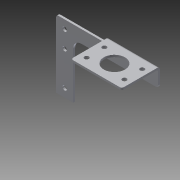
# Autodesk Inventor part: Circuit Breaker Mount
Saved by Autodesk Inventor 2013 (Build 170138000, 138)
## iProperties
Created: 2013-02-10
Part Number: Circuit Breaker Mount
Material: Aluminum 6061
Document SubType Name: Sheet Metal
Designer: Moses
Mass: 60.4905 g
Surface Area: 168.953 cm^2
Volume: 22.3212 cm^3
Density: 2.71 g/cm^3
Sheet Metal Rule: Default
Author: Moses
Autodesk Inventor part; units mm, degrees
ref_plane "YZ Plane" through (0, 0, 0) normal (1, 0, 0) x (0, 1, 0)
ref_plane "XZ Plane" through (0, 0, 0) normal (0, 1, 0) x (-1, 0, 0)
ref_plane "XY Plane" through (0, 0, 0) normal (0, 0, 1) x (1, 0, 0)
sketch "Sketch1" plane through (0, 0, 0) normal (0, 0, 1) x (1, 0, 0)
  line L0 (0, 0) -> (25.4, 0)
  line L1 (25.4, 0) -> (25.4, 50.8)
  line L2 (25.4, 50.8) -> (0, 50.8)
  line L3 (0, 50.8) -> (0, 0)
  line L4 (0, 25.4) -> (25.4, 25.4) construction
  line L5 (12.7, 38.1) -> (12.7, 12.7) construction
  circle A0 centre (12.7, 38.1) radius 3.302
  circle A1 centre (12.7, 12.7) radius 3.302
  line L6 (152.4, 50.8) -> (25.4, 50.8)
  line L7 (25.4, 31.75) -> (152.4, 31.75)
  line L8 (152.4, 31.75) -> (152.4, 50.8)
  line L9 (76.2, 50.8) -> (76.2, 53.975)
  line L10 (76.2, 53.975) -> (152.4, 53.975)
  line L11 (152.4, 53.975) -> (152.4, 50.8)
  line L12 (0, 0) -> (0, -50.8)
  line L13 (0, -50.8) -> (25.4, -50.8)
  line L14 (25.4, -50.8) -> (25.4, 0)
  line L15 (12.7, 12.7) -> (12.7, -38.1) construction
  circle A2 centre (12.7, -38.1) radius 3.302
  point P0 (12.7, 25.4)
  dimension "d0" = 25.4
  dimension "d2" = 6.604
  dimension "d3" = 6.604
  dimension "d4" = 50.8
  dimension "d5" = 25.4
  dimension "d6" = 127
  dimension "d7" = 19.05
  dimension "d8" = 76.2
  dimension "d9" = 3.175
  dimension "d32" = 50.8
  dimension "d33" = 6.604
  dimension "d34" = 12.7
  measures "d0" distance of L5.start L5.end
  measures "d2" diameter of A0
  measures "d3" diameter of A1
  measures "d4" distance of L2.end L0.start
  measures "d5" distance of L1.end L2.end
  measures "d6" distance of L6.start L1.end
  measures "d7" distance of L7.end L6.start
  measures "d8" distance of L9.end L10.end
  measures "d9" distance of L9.start L9.end
  measures "d32" distance of L15.start L15.end
  measures "d33" diameter of A2
  measures "d34" distance from line of L13 L15.end
extrude "Plate1" add sketch "Sketch1" along normal blind 3.048
sketch "Sketch2" plane through (76.2, 55.245, 4.318) normal (0, 1, 0) x (-1, 0, 0)
  line L0 (-76.2, 0) -> (0, 0)
  line L1 (0, 0) -> (0, 52.832)
  line L2 (0, 52.832) -> (-76.2, 52.832)
  line L3 (-76.2, 52.832) -> (-76.2, 0)
  constraints: 6 end point, 1 horizontal, 1 perpendicular, 1 vertical
edge flange "Flange1" height 57.15 angle 90 thickness 3.048 bend radius 1.27 thickness toward (0, 1, 0) relief straight relief width 3.048 relief depth 1.524 edges at (114.3, 53.975, 3.048) wall of the first edge with corners at (152.4, 55.245, 4.318) (76.2, 55.245, 4.318) (76.2, 55.245, 57.15) (152.4, 55.245, 57.15)
bend "Bend1"
corner "Corner1"
fillet "Corner Round1" radius 12.7 1 edges at (25.4, 31.75, 1.524)
fillet "Corner Round1" radius 3.175 5 edges at (0, 50.8, 1.524) (76.2, 56.769, 57.15) (152.4, 56.769, 57.15) (152.4, 31.75, 1.524) (76.2, 50.8, 1.524)
sketch "Sketch3" plane through (76.2, 58.293, 4.318) normal (0, 1, 0) x (1, 0, 0)
  line L0 (76.2, 0) -> (76.2, -49.657) projected
  line L1 (76.2, 0) -> (0, 0) projected
  circle A0 centre (66.675, -12.7) radius 3.302
  line L2 (0, -49.657) -> (0, 0) projected
  line L3 (73.025, -52.832) -> (3.175, -52.832) projected
  circle A1 centre (10.033, -39.37) radius 3.302
  line L4 (10.033, -39.37) -> (66.675, -39.37) construction
  line L5 (66.675, -39.37) -> (66.675, -12.7) construction
  line L6 (66.675, -12.7) -> (10.033, -12.7) construction
  line L7 (10.033, -12.7) -> (10.033, -39.37) construction
  circle A2 centre (10.033, -12.7) radius 3.302
  circle A3 centre (66.675, -39.37) radius 3.302
  line L8 (38.354, -12.7) -> (38.354, -39.37) construction
  circle A4 centre (38.354, -26.035) radius 15.875
  point P0 (-76.2, 4.318)
  dimension "d23" = 6.604
  dimension "d25" = 9.525
  dimension "d26" = 12.7
  dimension "d29" = 13.462
  dimension "d30" = 10.033
  dimension "d31" = 31.75
  constraints: 10 end point, 5 centre point, 3 equal radius, 3 midpoint, 2 coincident, 2 parallel, 1 horizontal, 1 perpendicular
  measures "d23" diameter of A0
  measures "d25" distance from line of L0 L5.end
  measures "d26" distance from line of L1 L5.end
  measures "d29" distance from line of L3 L4.start
  measures "d30" distance from line of L4.start L2
  measures "d31" diameter of A4
extrude "Cut1" cut sketch "Sketch3" against normal blind 3.048
equation "\"d27\" = Thickness"
equation "\"d11\" = BendReliefWidth"
equation "\"d12\" = BendReliefDepth"
equation "\"d13\" = MinimumRemnant"
equation "\"d14\" = BendRadius"
equation "\"d18\" = CornerReliefSize"
equation "\"d19\" = GapSize"
equation "\"d20\" = JacobiRadiusSize"
equation "\"BendRadius\" = Thickness"
equation "\"BendReliefWidth\" = Thickness"
equation "\"BendReliefDepth\" = 0.5 * Thickness"
equation "\"CornerReliefSize\" = 4 * Thickness"
equation "\"MinimumRemnant\" = 2 * Thickness"
equation "\"TransitionRadius\" = BendRadius"
equation "\"JacobiRadiusSize\" = BendRadius"
equation "\"GapSize\" = Thickness"
equation "\"d10\" = BendRadius"
equation "\"Thickness\" = 3.048"
body "Solid1"
